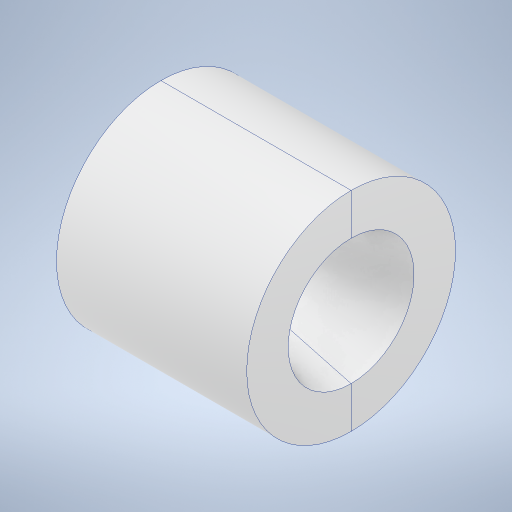
# Autodesk Inventor part: stainless steel space
Saved by Autodesk Inventor 2023 (Build 270158000, 158)
## iProperties
Created: 2022-09-19
Part Number: stainless steel space
Material: Aluminum 6061
Document SubType Name: Modeling
Designer: station
Density: 2.7 g/cm^3
Appearance: Aluminum - Flat
Author: station
Autodesk Inventor part; units mm, degrees
ref_plane "YZ Plane" through (0, 0, 0) normal (1, 0, 0) x (0, 1, 0)
ref_plane "XZ Plane" through (0, 0, 0) normal (0, 1, 0) x (-1, 0, 0)
sketch "Sketch3" plane through (0, 0, 0) normal (0, 0, 1) x (1, 0, 0)
  line L0 (0, 54.5) -> (192, 54.5)
  line L1 (254.7886, 18.124) -> (254.7886, 0) construction
  line L2 (192, 54.5) -> (254.7886, 18.124)
  line L3 (254.7886, 18.124) -> (325.1228, 36.97)
  line L4 (254.7886, 18.124) -> (254.7886, 43.3259) construction
  line L5 (0, 0) -> (254.7886, 0)
  line L6 (325.1228, 36.97) -> (325.1228, 0)
  line L7 (192, 54.5) -> (254.7886, 18.124)
  line L8 (325.1228, 0) -> (305.1228, 0)
  line L9 (-65.0246, 0) -> (390.1474, 0)
  line L10 (0, 57.5) -> (192, 57.5)
  line L11 (193.5039, 57.0958) -> (255.2149, 21.3441)
  line L12 (255.2149, 21.3441) -> (325.1228, 40.0758)
  line L13 (325.1228, 36.97) -> (325.1228, 40.0758)
  line L14 (0, 54.5) -> (0, 57.5)
  line L15 (193.5039, 57.0958) -> (192.8038, 57.5)
  line L16 (193.5039, 57.0958) -> (200.0085, 57.0958) construction
  line L17 (192, 57.5) -> (192.8038, 57.5)
  line L18 (325.1228, 40.0758) -> (325.1228, 57.5)
  line L19 (317.1228, 57.5) -> (317.1228, 37.9322)
  line L20 (325.1228, 0) -> (325.1228, 58.5)
  line L21 (317.1228, 58.5) -> (317.1228, 57.5)
  line L22 (317.1228, 58.5) -> (325.1228, 58.5)
  line L23 (317.1228, 58.5) -> (155.0777, 58.5)
  line L24 (192, 57.5) -> (192, 71.51)
  line L25 (192, 57.5) -> (206.01, 57.5) construction
  line L26 (192.8038, 57.5) -> (192.8038, 62.5821)
  line L27 (196.8038, 57.5) -> (196.8038, 62.5821)
  line L28 (196.8038, 57.5) -> (196.8038, 54.0674)
  line L29 (317.1228, 58.5) -> (303.4068, 58.5)
  line L30 (303.4068, 58.5) -> (303.4068, 12.5113)
  line L31 (324.864, 41.0418) -> (255.3571, 22.4174)
  line L32 (255.3571, 22.4174) -> (194.0045, 57.9615)
  line L33 (194.0045, 57.9615) -> (193.3038, 58.366)
  point P0 (327.1228, 40.0758)
  point P1 (254.7886, 31.9804)
  point P2 (325.1228, 59.5)
  point P3 (321.1228, 58.5)
  point P4 (196.8038, 56.3397)
  point P5 (303.4068, 35.2923)
  point P6 (196.8038, 58.5)
  dimension "d102" = 18.124
  dimension "d103" = 54.5
  dimension "d104" = 192
  dimension "d105" = 20
  dimension "d106" = 3
  dimension "d107" = 3
  dimension "d108" = 3
  dimension "d109" = 150
  dimension "d110" = 8
  dimension "d111" = 58.5
  dimension "d112" = 90
  dimension "d113" = 4
  dimension "d114" = 13.716
  dimension "d115" = 1
  constraints: 68 end point, 7 vertical, 5 horizontal, 4 point on line, 3 parallel, 3 perpendicular, 1 collinear, 1 midpoint, 2 other
  measures "d102" distance of L1.start L1.end
  measures "d103" distance from line of L5.start L0
  measures "d104" distance of L14.start L2.start
  measures "d105" distance of L6.end L8.end
  measures "d106" distance between parallel lines of L0 L10
  measures "d107" distance between parallel lines of L2 L11
  measures "d108" distance between parallel lines of L3 L12
  measures "d109" angle of L16 L15
  measures "d110" distance of L18.end L19.start
  measures "d111" distance from line of L8 point (321.123, 58.5)
  measures "d112" angle of L25 L24
  measures "d113" distance between parallel lines of L26 L27
  measures "d114" distance of L21.start L29.end
  measures "d115" distance between parallel lines of L11 L32
revolve "Revolution2" add sketch "Sketch3" angle 360 about axis through (-65.0246, 0, 0) along (1, 0, 0) contours L31 L32 L28 L27 L23 L30
ref_plane "Work Plane2" through (0, 0, 59.5) normal (0, 0, 1) x (1, 0, 0)
split body "Split6" result two bodies by plane through (0, 0, 0) normal (0, 0, 1) first body at (232.3382, -57.5604, 7.1275)
body "Solid3"
body "Solid4"
